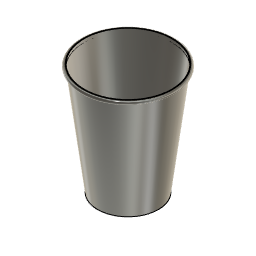
papercup v3 (Autodesk Fusion 360 design; units mm, degrees)
Autodesk Fusion 360 part; units mm, degrees
sketch "スケッチ1" plane through (0, 0, 0) normal (0, 0, 1) x (1, 0, 0)
  circle A0 centre (0, 0) radius 26
  circle A1 centre (0, 0) radius 25
  dimension "d1" = 52
  dimension "d8" = 50
  constraint coincident A0.centre A1.centre
  measures "d1" diameter of A0
  measures "d8" diameter of A1
ref_plane "作業平面1" through (0, 0, 95) normal (0, 0, 1) x (1, 0, 0)
sketch "スケッチ3" plane through (0, 0, 95) normal (0, 0, 1) x (1, 0, 0)
  circle A0 centre (0, 0) radius 40
  circle A1 centre (0, 0) radius 37.5
  circle A2 centre (0, 0) radius 38
  dimension "d6" = 80
  dimension "d7" = 75
  dimension "d11" = 76
  constraint coincident A0.centre A1.centre
  constraint concentric A0 A1
  constraint concentric A0 A2
  measures "d6" diameter of A0
  measures "d7" diameter of A1
  measures "d11" diameter of A2
ref_plane "作業平面2" through (0, 0, 5) normal (0, 0, 1) x (1, 0, 0)
sketch "スケッチ4" plane through (0, 0, 5) normal (0, 0, 1) x (1, 0, 0)
  circle A0 centre (0, 0) radius 25
  dimension "d10" = 50
  constraint coincident A0.centre origin
  measures "d10" diameter of A0
loft "ロフト1" add profiles "スケッチ1", "スケッチ3" section 1 contours A0 | A1 section 2 contours A1 | A2
loft "ロフト2" cut profiles "スケッチ1", "スケッチ4" section 1 contours A1 section 2
ref_plane "作業平面3" through (0, 0, 6) normal (0, 0, 1) x (1, 0, 0)
sketch "スケッチ5" plane through (0, 0, 6) normal (0, 0, 1) x (1, 0, 0)
  circle A0 centre (0, 0) radius 25
  dimension "d13" = 50
  constraint coincident A0.centre origin
  measures "d13" diameter of A0
ref_plane "作業平面4" through (0, 0, 93.5) normal (0, 0, 1) x (1, 0, 0)
sketch "スケッチ6" plane through (0, 0, 93.5) normal (0, 0, 1) x (1, 0, 0)
  circle A0 centre (0, 0) radius 38.5
  dimension "d15" = 77
  constraint coincident A0.centre origin
  measures "d15" diameter of A0
pipe "パイプ1" add diameter 3 path "スケッチ6" along A0
loft "ロフト3" cut profiles "スケッチ5", "スケッチ3" section 1 section 2 contours A1
